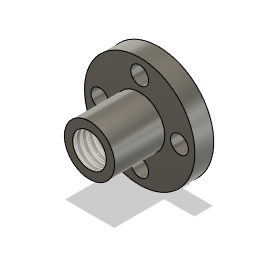
8mm Lead Screw Nut v1 (Autodesk Fusion 360 design; units mm, degrees)
Autodesk Fusion 360 part; units mm, degrees
sketch "Sketch2" plane through (0, 0, 0) normal (0, 0, 1) x (1, 0, 0)
  circle A0 centre (0, 0) radius 5.05
  circle A1 centre (0, 0) radius 11.1
  line L0 (-35, 0) -> (41.5964, 0) construction
  line L1 (0, 35) -> (0, -35) construction
  circle A2 centre (0, 8) radius 1.8
  circle A3 centre (8, 0) radius 1.8
  circle A4 centre (0, -8) radius 1.8
  circle A5 centre (-8, 0) radius 1.8
  circle A6 centre (0, 0) radius 8 construction
  circle A7 centre (0, 0) radius 4
  dimension "d1" = 10.1
  dimension "d2" = 22.2
  dimension "d3" = 3.6
  dimension "d4" = 3.6
  dimension "d5" = 3.6
  dimension "d6" = 3.6
  dimension "d7" = 16
  dimension "d13" = 8
  constraint coincident A0.centre A1.centre
  constraint horizontal L0
  constraint vertical L1
  constraint coincident L1 A2.centre
  constraint coincident L0 A3.centre
  constraint coincident L1 A4.centre
  constraint coincident L0 A5.centre
  constraint coincident A2.centre A6
  constraint coincident A3.centre A6
  constraint coincident A4.centre A6
  constraint coincident A5.centre A6
  measures "d1" diameter of A0
  measures "d2" diameter of A1
  measures "d3" diameter of A2
  measures "d4" diameter of A3
  measures "d5" diameter of A4
  measures "d6" diameter of A5
  measures "d7" diameter of A6
  measures "d13" diameter of A7
extrude "Extrude1" add sketch "Sketch2" along normal blind 15.5 contours A0 | A7
extrude "Extrude2" add sketch "Sketch2" along normal blind 3.8 from surface at 1.6 contours A1
extrude "Extrude3" cut sketch "Sketch2" along normal up to surface (15.5 mm away) contours A7
thread "Thread1" "ISO Metric profile 8.0 M8x1.25 6H" major diameter 8.17 minor diameter 6.7795 pitch 1.25 angle 60 resizes the face on face at (3.995, -0.1994, 10.3333)
